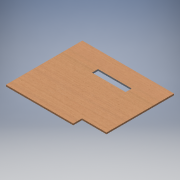
# Autodesk Inventor part: cote
Saved by Autodesk Inventor 2019 (Build 230136000, 136)
## iProperties
Created: 2020-02-15
Part Number: cote
Material: Generic
Document SubType Name: Modeling
Designer: franc
Density: 1 g/cm^3
Appearance: Default
Author: franc
Autodesk Inventor part; units mm, degrees
ref_plane "YZ Plane" through (0, 0, 0) normal (1, 0, 0) x (0, 1, 0)
ref_plane "XZ Plane" through (0, 0, 0) normal (0, 1, 0) x (-1, 0, 0)
ref_plane "XY Plane" through (0, 0, 0) normal (0, 0, 1) x (1, 0, 0)
sketch "Esquisse1" plane through (0, 0, 0) normal (0, 1, 0) x (-1, 0, 0)
  line L0 (100.2268, 65.494) -> (-119.7732, 65.494)
  line L1 (-199.7732, 36.494) -> (-199.7732, -184.506)
  line L2 (-199.7732, -184.506) -> (100.2268, -184.506)
  line L3 (100.2268, -184.506) -> (100.2268, 65.494)
  line L4 (-119.7732, 65.494) -> (-119.7732, 36.494)
  line L5 (-119.7732, 36.494) -> (-199.7732, 36.494)
  point P0 (0, 0)
  dimension "d0" = 250
  dimension "d1" = 300
  dimension "d4" = 221
  dimension "d5" = 80
  constraints: 12 end point, 2 parallel, 2 perpendicular, 1 horizontal, 1 vertical
  measures "d0" distance of L2.end L0.start
  measures "d1" distance of L1.end L2.end
  measures "d4" distance between parallel lines of L2 L5
  measures "d5" distance between parallel lines of L1 L4
extrude "Extrusion1" add sketch "Esquisse1" along normal blind 5
sketch "Esquisse2" plane through (0, 5, 0) normal (0, 1, 0) x (1, 0, 0)
  line L0 (6.299, 109.506) -> (116.299, 109.506)
  line L1 (116.299, 109.506) -> (116.299, 129.506)
  line L2 (116.299, 129.506) -> (6.299, 129.506)
  line L3 (6.299, 129.506) -> (6.299, 109.506)
  line L4 (199.7732, 184.506) -> (-100.2268, 184.506) projected
  point P0 (0, 0)
  dimension "d6" = 20
  dimension "d7" = 110
  dimension "d8" = 55
  constraints: 8 end point, 2 parallel, 1 horizontal, 1 perpendicular
  measures "d6" distance of L2.end L0.start
  measures "d7" distance of L1.end L2.end
  measures "d8" distance between parallel lines of L4 L2
extrude "Extrusion2" cut sketch "Esquisse2" against normal through all
